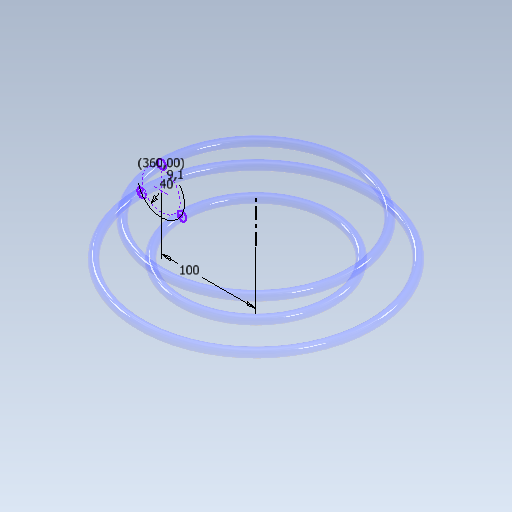
# Autodesk Inventor part: трубочки_мозговорота
Saved by Autodesk Inventor 2021.1 (Build 251245010, 245A)
## iProperties
Created: 2022-11-18
Part Number: трубочки_мозговорота
Material: Типовые
Document SubType Name: Modeling
Designer: zmoze
Density: 1 g/cm^3
Appearance: Прозрачный — синий
Author: zmoze
Autodesk Inventor part; units mm, degrees
ref_plane "YZ Plane" through (0, 0, 0) normal (1, 0, 0) x (0, 1, 0)
ref_plane "XZ Plane" through (0, 0, 0) normal (0, 1, 0) x (-1, 0, 0)
ref_plane "XY Plane" through (0, 0, 0) normal (0, 0, 1) x (1, 0, 0)
sketch "Эскиз1" plane through (0, 0, 0) normal (0, 0, 1) x (1, 0, 0)
  circle A0 centre (-100, 24.55) radius 4.55
  circle A1 centre (-121.2609, -12.275) radius 4.55
  circle A2 centre (-78.7391, -12.275) radius 4.55
  line L0 (0, 0) -> (0, 43.5708)
  circle A3 centre (-100, 0) radius 20 construction
  line L1 (-100, 0) -> (-100, 24.55) construction
  dimension "d1" = 9.1
  dimension "d10" = 360
  dimension "d14" = 40
  dimension "d15" = 100
  constraints: 4 centre point, 4 end point, 3 tangent, 2 vertical, 7 other
  measures "d1" diameter of A0
  measures "d14" diameter of A3
  measures "d15" distance of L1.start L0.start
revolve "Вращение1" add sketch "Эскиз1" angle 360 about axis through (0, 0, 0) along (0, 1, 0)
